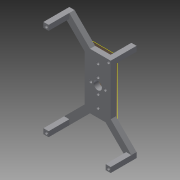
# Autodesk Inventor part: Face
Saved by Autodesk Inventor 2015 (Build 190159000, 159)
## iProperties
Created: 2015-03-18
Part Number: Face
Material: Generic
Document SubType Name: Modeling
Designer: ChristopherEvan
Density: 1 g/cm^3
Appearance: Default
Author: ChristopherEvan
Autodesk Inventor part; units mm, degrees
ref_plane "YZ Plane" through (0, 0, 0) normal (1, 0, 0) x (0, 1, 0)
ref_plane "XZ Plane" through (0, 0, 0) normal (0, 1, 0) x (-1, 0, 0)
ref_plane "XY Plane" through (0, 0, 0) normal (0, 0, 1) x (1, 0, 0)
ref_plane "Work Plane1" through (0, 0, 35) normal (0, 0, 1) x (1, 0, 0)
sketch "Sketch1" plane through (0, 0, 35) normal (0, 0, 1) x (1, 0, 0)
  circle A0 centre (12.5, 45.6) radius 1.5 projected
  circle A1 centre (19.5, 27) radius 1.5 projected
  circle A2 centre (5.5, 27) radius 1.5 projected
  circle A3 centre (12.5, 20) radius 1.5 projected
  circle A4 centre (12.5, 34) radius 1.5 projected
  circle A5 centre (12.5, 8.4) radius 1.5 projected
  circle A6 centre (12.5, 27) radius 4 projected
  line L0 (0, 0) -> (25, 0) projected
  line L1 (25, 0) -> (25, 54) projected
  line L2 (0, 54) -> (25, 54) projected
  line L3 (0, 0) -> (0, 54) projected
  line L4 (25, 54) -> (0, 54)
  line L5 (0, 54) -> (0, 0)
  line L6 (0, 0) -> (25, 0)
  line L7 (25, 0) -> (25, 54)
  circle A7 centre (12.5, 45.6) radius 1.5
  circle A8 centre (12.5, 27) radius 4
  circle A9 centre (19.5, 27) radius 1.5
  circle A10 centre (12.5, 34) radius 1.5
  circle A11 centre (12.5, 20) radius 1.5
  circle A12 centre (5.5, 27) radius 1.5
  circle A13 centre (12.5, 8.4) radius 1.5
  constraints: 8 end point, 7 centre point, 7 coincident, 7 concentric, 2 parallel, 1 horizontal, 1 perpendicular
extrude "Extrusion1" add sketch "Sketch1" along normal blind 5
sketch "Sketch4" plane through (0, 0, 40) normal (0, 0, 1) x (1, 0, 0)
  line L0 (25, 54) -> (0, 54) projected
  line L1 (0, 54) -> (0, 0) projected
  circle A0 centre (12.5, 45.6) radius 1.5 projected
  line L2 (25, 0) -> (25, 54) projected
  line L3 (0, 0) -> (25, 0) projected
  line L4 (25, 54) -> (45, 54)
  line L5 (45, 54) -> (45, 74)
  line L6 (45, 74) -> (25, 74)
  line L7 (25, 74) -> (25, 54)
  line L8 (0, 54) -> (-20, 54)
  line L9 (-20, 54) -> (-20, 74)
  line L10 (-20, 74) -> (0, 74)
  line L11 (0, 74) -> (0, 54)
  line L12 (25, 0) -> (45, 0)
  line L13 (45, 0) -> (45, -20)
  line L14 (45, -20) -> (25, -20)
  line L15 (25, -20) -> (25, 0)
  line L16 (0, 0) -> (-20, 0)
  line L17 (-20, 0) -> (-20, -20)
  line L18 (-20, -20) -> (0, -20)
  line L19 (0, -20) -> (0, 0)
  line L20 (-20, 74) -> (-15, 74)
  line L21 (-15, 74) -> (-15, 69)
  line L22 (-15, 69) -> (-20, 69)
  line L23 (-20, 69) -> (-20, 74)
  line L24 (45, 74) -> (40, 74)
  line L25 (40, 74) -> (40, 69)
  line L26 (40, 69) -> (45, 69)
  line L27 (45, 69) -> (45, 74)
  line L28 (45, -20) -> (40, -20)
  line L29 (40, -20) -> (40, -15)
  line L30 (40, -15) -> (45, -15)
  line L31 (45, -15) -> (45, -20)
  line L32 (-20, -20) -> (-15, -20)
  line L33 (-15, -20) -> (-15, -15)
  line L34 (-15, -15) -> (-20, -15)
  line L35 (-20, -15) -> (-20, -20)
  line L36 (0, 0) -> (5, 0)
  line L37 (5, 0) -> (5, 5)
  line L38 (5, 5) -> (0, 5)
  line L39 (0, 5) -> (0, 0)
  line L40 (25, 0) -> (20, 0)
  line L41 (20, 0) -> (20, 5)
  line L42 (20, 5) -> (25, 5)
  line L43 (25, 5) -> (25, 0)
  line L44 (25, 54) -> (20, 54)
  line L45 (20, 54) -> (20, 49)
  line L46 (20, 49) -> (25, 49)
  line L47 (25, 49) -> (25, 54)
  line L48 (0, 54) -> (5, 54)
  line L49 (5, 54) -> (5, 49)
  line L50 (5, 49) -> (0, 49)
  line L51 (0, 49) -> (0, 54)
  line L52 (0, 5) -> (-20, -15)
  line L53 (5, 0) -> (-15, -20)
  line L54 (20, 0) -> (40, -20)
  line L55 (25, 5) -> (45, -15)
  line L56 (-20, 69) -> (0, 49)
  line L57 (-15, 74) -> (5, 54)
  line L58 (40, 74) -> (20, 54)
  line L59 (45, 69) -> (25, 49)
  circle A1 centre (-17.5, 71.5) radius 1.5
  circle A2 centre (42.5, 71.5) radius 1.5
  circle A3 centre (-17.5, -17.5) radius 1.5
  circle A4 centre (42.5, -17.5) radius 1.5
  dimension "d16" = 20
  dimension "d17" = 20
  dimension "d18" = 20
  dimension "d19" = 20
  dimension "d20" = 20
  dimension "d21" = 20
  dimension "d22" = 20
  dimension "d23" = 20
  dimension "d24" = 5
  dimension "d25" = 5
  dimension "d26" = 5
  dimension "d27" = 5
  dimension "d28" = 5
  dimension "d29" = 5
  dimension "d30" = 5
  dimension "d31" = 5
  dimension "d32" = 5
  dimension "d33" = 5
  dimension "d34" = 5
  dimension "d35" = 5
  dimension "d36" = 5
  dimension "d37" = 5
  dimension "d38" = 5
  dimension "d39" = 5
  dimension "d40" = 3
  constraints: 112 end point, 24 parallel, 12 horizontal, 12 perpendicular, 4 centre point
  measures "d16" distance of L6.end L5.end
  measures "d17" distance of L5.end L4.end
  measures "d18" distance of L9.end L10.end
  measures "d19" distance of L8.end L9.end
  measures "d20" distance of L13.end L14.end
  measures "d21" distance of L12.end L13.end
  measures "d22" distance of L18.end L17.end
  measures "d23" distance of L17.end L16.end
  measures "d24" distance of L21.end L22.end
  measures "d25" distance of L20.end L21.end
  measures "d26" distance of L26.end L25.end
  measures "d27" distance of L25.end L24.end
  measures "d28" distance of L29.end L30.end
  measures "d29" distance of L28.end L29.end
  measures "d30" distance of L34.end L33.end
  measures "d31" distance of L33.end L32.end
  measures "d32" distance of L38.end L37.end
  measures "d33" distance of L37.end L36.end
  measures "d34" distance of L41.end L42.end
  measures "d35" distance of L40.end L41.end
  measures "d36" distance of L46.end L45.end
  measures "d37" distance of L45.end L44.end
  measures "d38" distance of L49.end L50.end
  measures "d39" distance of L48.end L49.end
  measures "d40" diameter of A1
extrude "Extrusion3" add sketch "Sketch4" against normal blind 5 contours L2 L46 L45 L0 | L4 L59 L2 | L7 L58 L25 L26 L59 L4 | L0 L58 L7 | L49 L50 L1 L0 | L0 L11 L57 | L55 L12 L2 | L2 L3 L41 L42 | L26 L25 L6 L5 | L1 L56 L8 | L8 L56 L22 L21 L57 L11 | L15 L54 L3 | L12 L55 L30 L29 L54 L15 | L21 L22 L9 L10 | L13 L14 L29 L30 | L38 L37 L3 L1 | L1 L16 L52 | L53 L19 L3 | L19 L53 L33 L34 L52 L16 | L34 L33 L18 L17
sketch "Sketch5" plane through (0, 0, 40) normal (0, 0, 1) x (1, 0, 0)
  line L0 (-20, -20) -> (-15, -20) projected
  line L1 (-20, -15) -> (-20, -20) projected
  circle A0 centre (-17.5, -17.5) radius 1.5 projected
  circle A1 centre (-17.5, 71.5) radius 1.5 projected
  line L2 (-20, 74) -> (-20, 69) projected
  line L3 (-15, 74) -> (-20, 74) projected
  line L4 (45, 74) -> (40, 74) projected
  line L5 (45, 69) -> (45, 74) projected
  circle A2 centre (42.5, 71.5) radius 1.5 projected
  circle A3 centre (42.5, -17.5) radius 1.5 projected
  line L6 (40, -20) -> (45, -20) projected
  line L7 (45, -20) -> (45, -15) projected
  line L8 (-20, -20) -> (-15, -20)
  line L9 (-15, -20) -> (-15, -15)
  line L10 (-15, -15) -> (-20, -15)
  line L11 (-20, -15) -> (-20, -20)
  circle A4 centre (-17.5, -17.5) radius 1.5
  circle A5 centre (-17.5, 71.5) radius 1.5
  circle A6 centre (42.5, 71.5) radius 1.5
  circle A7 centre (42.5, -17.5) radius 1.5
  line L12 (40, -20) -> (45, -20)
  line L13 (45, -20) -> (45, -15)
  line L14 (45, -15) -> (40, -15)
  line L15 (40, -15) -> (40, -20)
  line L16 (45, 74) -> (40, 74)
  line L17 (40, 74) -> (40, 69)
  line L18 (40, 69) -> (45, 69)
  line L19 (45, 69) -> (45, 74)
  line L20 (-20, 69) -> (-15, 69)
  line L21 (-15, 69) -> (-15, 74)
  line L22 (-15, 74) -> (-20, 74)
  line L23 (-20, 74) -> (-20, 69)
  point P0 (0, 0)
  constraints: 32 end point, 8 parallel, 4 centre point, 4 coincident, 4 concentric, 4 horizontal, 4 perpendicular, 1 point on line
extrude "Extrusion4" add sketch "Sketch5" along normal blind 20
body "Solid1"
